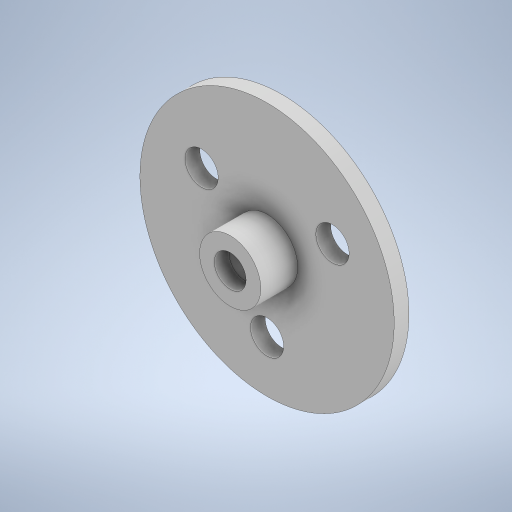
# Autodesk Inventor part: na magnes
Saved by Autodesk Inventor 2023 (Build 270158000, 158)
## iProperties
Created: 2023-04-11
Part Number: na magnes
Material: Ogólny
Document SubType Name: Modeling
Designer: Kamil
Density: 1 g/cm^3
Appearance: Domyślna
Author: Kamil
Autodesk Inventor part; units mm, degrees
ref_plane "YZ Plane" through (0, 0, 0) normal (1, 0, 0) x (0, 1, 0)
ref_plane "XZ Plane" through (0, 0, 0) normal (0, 1, 0) x (-1, 0, 0)
ref_plane "XY Plane" through (0, 0, 0) normal (0, 0, 1) x (1, 0, 0)
sketch "Szkic1" plane through (0, 0, 0) normal (0, 0, 1) x (1, 0, 0)
  circle A0 centre (-8.8768, 43) radius 2 projected
  circle A1 centre (8.8768, 43) radius 2 projected
  circle A2 centre (0, 27.625) radius 2 projected
  line L0 (20.7693, 46.5287) -> (55.6245, -37.125) projected
  arc A3 (20.7693, 46.5287) -> (-20.7693, 46.5287) centre (0, 37.875) ccw projected
  line L1 (-55.6245, -37.125) -> (-20.7693, 46.5287) projected
  line L2 (-55.6245, -63.375) -> (-55.6245, -37.125) projected
  line L3 (55.6245, -63.375) -> (-55.6245, -63.375) projected
  line L4 (55.6245, -37.125) -> (55.6245, -63.375) projected
  circle A4 centre (-50, -53.375) radius 2.75 projected
  circle A5 centre (50, -53.375) radius 2.75 projected
  circle A6 centre (-25, -45.375) radius 2.75 projected
  circle A7 centre (25, -45.375) radius 2.75 projected
  circle A8 centre (0, -53.375) radius 2.75 projected
  circle A9 centre (0, 37.875) radius 17.2375
  circle A10 centre (0, 37.875) radius 2.1667
  point P0 (0, 0)
  constraints: 2 centre point, 2 coincident
extrude "Wyciągnięcie proste1" add sketch "Szkic1" along normal blind 2.54 contours A9
sketch "Szkic2" plane through (0, 37.875, 2.54) normal (0, 0, 1) x (1, 0, 0)
  circle A0 centre (0, 0) radius 17.2375 projected
  circle A1 centre (0, 0) radius 2.1667 projected
  circle A2 centre (0, -10.25) radius 2 projected
  circle A3 centre (8.8768, 5.125) radius 2 projected
  circle A4 centre (-8.8768, 5.125) radius 2 projected
  point P0 (0, -37.875)
extrude "Wyciągnięcie proste2" cut sketch "Szkic2" against normal blind 0.54
sketch "Szkic3" plane through (0, 37.875, 2) normal (0, 0, 1) x (1, 0, 0)
  circle A0 centre (0, 0) radius 17.2375 projected
  circle A1 centre (-8.8768, 5.125) radius 2 projected
  circle A2 centre (8.8768, 5.125) radius 2 projected
  circle A3 centre (0, -10.25) radius 2 projected
  circle A4 centre (0, 0) radius 2.1667 projected
  point P0 (0, -37.875)
extrude "Wyciągnięcie proste3" add sketch "Szkic3" against normal up to surface (2 mm away) contours A4
sketch "Szkic4" plane through (0, 37.875, 2) normal (0, 0, 1) x (1, 0, 0)
  circle A0 centre (0, 0) radius 17.2375 projected
  circle A1 centre (-8.8768, 5.125) radius 2 projected
  circle A2 centre (8.8768, 5.125) radius 2 projected
  circle A3 centre (0, -10.25) radius 2 projected
  circle A4 centre (0, 0) radius 2.15
  line L0 (2.15, 0) -> (4.15, 0)
  circle A5 centre (0, 0) radius 4.15
  point P0 (0, -37.875)
  dimension "d6" = 4.3
  dimension "d7" = 2
  constraints: 2 coincident, 2 end point, 2 horizontal alignment, 1 horizontal, 4 other
  measures "d7" distance of L0.start L0.end
extrude "Wyciągnięcie proste4" add sketch "Szkic4" along normal blind 5 contours A5
sketch "Szkic5" plane through (0, 37.875, 2) normal (0, 0, 1) x (1, 0, 0)
  circle A0 centre (0, 0) radius 2.15 projected
  point P0 (0, -37.875)
extrude "Wyciągnięcie proste5" add sketch "Szkic5" along normal blind 3
sketch "Szkic6" plane through (0, 37.875, 2) normal (0, 0, 1) x (1, 0, 0)
  circle A0 centre (0, 0) radius 17.2375 projected
  circle A1 centre (-8.8768, 5.125) radius 2 projected
  circle A2 centre (8.8768, 5.125) radius 2 projected
  circle A3 centre (0, -10.25) radius 2 projected
  circle A4 centre (0, -10.25) radius 2.25
  circle A5 centre (-8.8768, 5.125) radius 2.25
  circle A6 centre (8.8768, 5.125) radius 2.25
  point P0 (0, -37.875)
  dimension "d16" = 4.5
  dimension "d17" = 4.5
  dimension "d18" = 4.5
  constraints: 3 centre point, 3 coincident
  measures "d16" diameter of A4
  measures "d17" diameter of A5
  measures "d18" diameter of A6
extrude "Wyciągnięcie proste6" cut sketch "Szkic6" against normal through all contours A1 | A2 | A3 | A4 | A5 | A6
